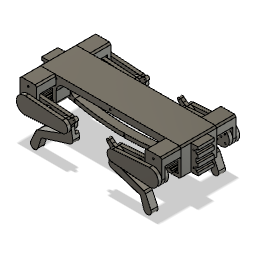
forGazebo v6 (Autodesk Fusion 360 design; units mm, degrees)
Autodesk Fusion 360 part; units mm, degrees
sketch "Sketch1" plane through (0, 0, 0) normal (0, 0, 1) x (1, 0, 0)
  arc A0 (83.6533, -28.925) -> (83.3871, -29.3635) centre (83.6533, -29.225) ccw
  arc A1 (81.6129, -29.3635) -> (83.3871, -29.3635) centre (82.5, -29.825) ccw
  arc A2 (81.6129, -29.3635) -> (81.3467, -28.925) centre (81.3467, -29.225) ccw
  arc A3 (-81.3467, -28.925) -> (-81.6129, -29.3635) centre (-81.3467, -29.225) ccw
  line L0 (-81.3467, -28.925) -> (-79, -28.925)
  arc A4 (-83.3871, -29.3635) -> (-83.6533, -28.925) centre (-83.6533, -29.225) ccw
  line L1 (-86, -28.925) -> (-83.6533, -28.925)
  line L2 (-86, -28.175) -> (-86, -28.925)
  line L3 (-86, -27.675) -> (-86, -28.175)
  line L4 (-79, -28.175) -> (-79, -27.675)
  line L5 (-79, -28.925) -> (-79, -28.175)
  line L6 (79, -28.175) -> (79, -28.925)
  line L7 (79, -27.675) -> (79, -28.175)
  line L8 (83.6533, -28.925) -> (86, -28.925)
  line L9 (86, -28.175) -> (86, -27.675)
  line L10 (86, -28.925) -> (86, -28.175)
  line L11 (79, -28.925) -> (81.3467, -28.925)
  line L12 (-79, -27.675) -> (-77.05, -27.675)
  line L13 (-87.95, -27.675) -> (-86, -27.675)
  line L14 (86, -27.675) -> (87.95, -27.675)
  line L15 (77.05, -27.675) -> (79, -27.675)
  line L16 (102.4, -1.585) -> (100.1, -1.585)
  arc A5 (-83.3871, -29.3635) -> (-81.6129, -29.3635) centre (-82.5, -29.825) ccw
  circle A6 centre (-71.05, 0) radius 1
  circle A7 centre (71.05, 0) radius 1
  circle A8 centre (-65.2986, -31.4552) radius 1
  circle A9 centre (65.2986, -31.4552) radius 1
  circle A10 centre (0, -38.7099) radius 1
  circle A11 centre (-97.3, -24.2) radius 1
  circle A12 centre (-97.3, -4.2) radius 1
  circle A13 centre (97.3, -24.2) radius 1
  circle A14 centre (97.3, -4.2) radius 1
  line L17 (-60, -4.275) -> (-50, -4.275)
  line L18 (-50, 4.275) -> (-60, 4.275)
  line L19 (-85, -4.275) -> (-80, -4.275)
  line L20 (-80, 4.275) -> (-85, 4.275)
  spline S0 degree 3 poles (-83.5, -2.125) (-83.5, -1.9978) (-83.4743, -1.8633) (-83.3718, -1.6174) (-83.2951, -1.5059) (-83.1192, -1.3299) (-83.0076, -1.2532) (-82.7616, -1.1507) (-82.6271, -1.125) (-82.3729, -1.125) (-82.2384, -1.1507) (-81.9924, -1.2532) (-81.8808, -1.3299) (-81.7049, -1.5059) (-81.6282, -1.6174) (-81.5257, -1.8633) (-81.5, -1.9978) (-81.5, -2.2522) (-81.5257, -2.3867) (-81.6282, -2.6326) (-81.7049, -2.7441) (-81.8808, -2.9201) (-81.9924, -2.9968) (-82.2384, -3.0993) (-82.3729, -3.125) (-82.6271, -3.125) (-82.7616, -3.0993) (-83.0076, -2.9968) (-83.1192, -2.9201) (-83.2951, -2.7441) (-83.3718, -2.6326) (-83.4743, -2.3867) (-83.5, -2.2522) (-83.5, -2.125) knots 0 0 0 0 0.038156 0.038156 0.076312 0.076312 0.114429 0.114429 0.152546 0.152546 0.190663 0.190663 0.22878 0.22878 0.266936 0.266936 0.305092 0.305092 0.343248 0.343248 0.381403 0.381403 0.41952 0.41952 0.457638 0.457638 0.495755 0.495755 0.533872 0.533872 0.572028 0.572028 0.610183 0.610183 0.610183 0.610183
  line L21 (80, -4.275) -> (85, -4.275)
  line L22 (85, 4.275) -> (80, 4.275)
  spline S1 degree 3 poles (81.5, -2.125) (81.5, -1.9978) (81.5257, -1.8633) (81.6282, -1.6174) (81.7049, -1.5059) (81.8808, -1.3299) (81.9924, -1.2532) (82.2384, -1.1507) (82.3729, -1.125) (82.6271, -1.125) (82.7616, -1.1507) (83.0076, -1.2532) (83.1192, -1.3299) (83.2951, -1.5059) (83.3718, -1.6174) (83.4743, -1.8633) (83.5, -1.9978) (83.5, -2.2522) (83.4743, -2.3867) (83.3718, -2.6326) (83.2951, -2.7441) (83.1192, -2.9201) (83.0076, -2.9968) (82.7616, -3.0993) (82.6271, -3.125) (82.3729, -3.125) (82.2384, -3.0993) (81.9924, -2.9968) (81.8808, -2.9201) (81.7049, -2.7441) (81.6282, -2.6326) (81.5257, -2.3867) (81.5, -2.2522) (81.5, -2.125) knots 0 0 0 0 0.038156 0.038156 0.076312 0.076312 0.114429 0.114429 0.152546 0.152546 0.190663 0.190663 0.22878 0.22878 0.266936 0.266936 0.305092 0.305092 0.343248 0.343248 0.381403 0.381403 0.41952 0.41952 0.457638 0.457638 0.495755 0.495755 0.533872 0.533872 0.572028 0.572028 0.610183 0.610183 0.610183 0.610183
  line L23 (50, -4.275) -> (60, -4.275)
  line L24 (60, 4.275) -> (50, 4.275)
  line L25 (-85, -4.275) -> (-87.95, -4.275)
  line L26 (80, -4.275) -> (77.05, -4.275)
  line L27 (87.95, -4.275) -> (85, -4.275)
  line L28 (-80, 4.275) -> (-60, 4.275)
  line L29 (-91.5, 4.275) -> (-85, 4.275)
  line L30 (85, 4.275) -> (91.5, 4.275)
  line L31 (60, 4.275) -> (80, 4.275)
  line L32 (-50, 4.275) -> (50, 4.275)
  line L33 (61.05, -4.275) -> (60, -4.275)
  line L34 (-60, -4.275) -> (-61.05, -4.275)
  line L35 (50, -4.275) -> (-50, -4.275)
  circle A15 centre (0, 0) radius 1
  arc A16 (-88.95, -26.675) -> (-87.95, -27.675) centre (-88.95, -27.675) ccw
  arc A17 (-87.95, -4.275) -> (-88.95, -5.275) centre (-88.95, -4.275) ccw
  line L36 (-77.05, -4.275) -> (-80, -4.275)
  arc A18 (-76.05, -5.275) -> (-77.05, -4.275) centre (-76.05, -4.275) ccw
  line L37 (-88.95, -5.275) -> (-88.95, -26.675)
  line L38 (-76.05, -26.675) -> (-76.05, -5.275)
  arc A19 (-77.05, -27.675) -> (-76.05, -26.675) centre (-76.05, -27.675) ccw
  arc A20 (76.05, -26.675) -> (77.05, -27.675) centre (76.05, -27.675) ccw
  arc A21 (77.05, -4.275) -> (76.05, -5.275) centre (76.05, -4.275) ccw
  arc A22 (88.95, -5.275) -> (87.95, -4.275) centre (88.95, -4.275) ccw
  line L39 (76.05, -5.275) -> (76.05, -26.675)
  line L40 (88.95, -26.675) -> (88.95, -5.275)
  arc A23 (87.95, -27.675) -> (88.95, -26.675) centre (88.95, -27.675) ccw
  arc A24 (71.05, -14.275) -> (61.05, -4.275) centre (61.05, -14.275) ccw
  line L41 (71.05, -21.1412) -> (71.05, -14.275)
  arc A25 (64.7498, -29.0162) -> (71.05, -21.1412) centre (62.9781, -21.1412) ccw
  arc A26 (-64.7498, -29.0162) -> (64.7498, -29.0162) centre (0, 258.7901) ccw
  arc A27 (-71.05, -21.1412) -> (-64.7498, -29.0162) centre (-62.9781, -21.1412) ccw
  line L42 (-71.05, -14.275) -> (-71.05, -21.1412)
  arc A28 (-61.05, -4.275) -> (-71.05, -14.275) centre (-61.05, -14.275) ccw
  line L43 (91.5, -32.675) -> (76.8218, -32.675)
  arc A29 (76.8218, -32.675) -> (65.8473, -33.8943) centre (76.8218, -82.675) ccw
  arc A30 (-65.8473, -33.8943) -> (65.8473, -33.8943) centre (0, 258.7901) ccw
  arc A31 (-65.8473, -33.8943) -> (-76.8218, -32.675) centre (-76.8218, -82.675) ccw
  line L44 (-76.8218, -32.675) -> (-91.5, -32.675)
  line L45 (102.9, 2.275) -> (102.9, -1.585)
  line L46 (102.9, -1.585) -> (102.4, -1.585)
  line L47 (93.5, 2.275) -> (102.9, 2.275)
  line L48 (91.5, 4.275) -> (93.5, 2.275)
  line L49 (-93.5, 2.275) -> (-91.5, 4.275)
  line L50 (-102.9, 2.275) -> (-93.5, 2.275)
  line L51 (-102.9, -1.585) -> (-102.9, 2.275)
  line L52 (-100.1, -1.585) -> (-102.9, -1.585)
  line L53 (-100.1, -6.815) -> (-100.1, -1.585)
  line L54 (-102.9, -6.815) -> (-100.1, -6.815)
  line L55 (-102.9, -11.585) -> (-102.9, -6.815)
  line L56 (-100.1, -11.585) -> (-102.9, -11.585)
  line L57 (-100.1, -16.815) -> (-100.1, -11.585)
  line L58 (-102.9, -16.815) -> (-100.1, -16.815)
  line L59 (-102.9, -21.585) -> (-102.9, -16.815)
  line L60 (-100.1, -21.585) -> (-102.9, -21.585)
  line L61 (-100.1, -26.815) -> (-100.1, -21.585)
  line L62 (-102.9, -26.815) -> (-100.1, -26.815)
  line L63 (-102.9, -30.675) -> (-102.9, -26.815)
  line L64 (-93.5, -30.675) -> (-102.9, -30.675)
  line L65 (-91.5, -32.675) -> (-93.5, -30.675)
  line L66 (93.5, -30.675) -> (91.5, -32.675)
  line L67 (102.9, -30.675) -> (93.5, -30.675)
  line L68 (102.9, -26.815) -> (102.9, -30.675)
  line L69 (100.1, -26.815) -> (102.9, -26.815)
  line L70 (100.1, -21.585) -> (100.1, -26.815)
  line L71 (102.9, -21.585) -> (100.1, -21.585)
  line L72 (102.9, -16.815) -> (102.9, -21.585)
  line L73 (100.1, -16.815) -> (102.9, -16.815)
  line L74 (100.1, -11.585) -> (100.1, -16.815)
  line L75 (102.9, -11.585) -> (100.1, -11.585)
  line L76 (102.9, -6.815) -> (102.9, -11.585)
  line L77 (100.1, -6.815) -> (102.9, -6.815)
  line L78 (100.1, -1.585) -> (100.1, -6.815)
  arc A32 (-81.3467, -28.925) -> (-81.6129, -29.3635) centre (-81.3467, -29.225) ccw
  arc A33 (-83.3871, -29.3635) -> (-81.6129, -29.3635) centre (-82.5, -29.825) ccw
  arc A34 (-83.3871, -29.3635) -> (-83.6533, -28.925) centre (-83.6533, -29.225) ccw
  line L79 (-83.6533, -28.925) -> (-86, -28.925)
  line L80 (-86, -28.925) -> (-86, -27.675)
  line L81 (-86, -27.675) -> (-87.95, -27.675)
  arc A35 (-88.95, -26.675) -> (-87.95, -27.675) centre (-88.95, -27.675) ccw
  line L82 (-88.95, -26.675) -> (-88.95, -5.275)
  arc A36 (-87.95, -4.275) -> (-88.95, -5.275) centre (-88.95, -4.275) ccw
  line L83 (-87.95, -4.275) -> (-77.05, -4.275)
  arc A37 (-76.05, -5.275) -> (-77.05, -4.275) centre (-76.05, -4.275) ccw
  line L84 (-76.05, -5.275) -> (-76.05, -26.675)
  arc A38 (-77.05, -27.675) -> (-76.05, -26.675) centre (-76.05, -27.675) ccw
  line L85 (-77.05, -27.675) -> (-79, -27.675)
  line L86 (-79, -27.675) -> (-79, -28.925)
  line L87 (-79, -28.925) -> (-81.3467, -28.925)
  arc A39 (83.6533, -28.925) -> (83.3871, -29.3635) centre (83.6533, -29.225) ccw
  arc A40 (81.6129, -29.3635) -> (83.3871, -29.3635) centre (82.5, -29.825) ccw
  arc A41 (81.6129, -29.3635) -> (81.3467, -28.925) centre (81.3467, -29.225) ccw
  line L88 (81.3467, -28.925) -> (79, -28.925)
  line L89 (79, -28.925) -> (79, -27.675)
  line L90 (79, -27.675) -> (77.05, -27.675)
  arc A42 (76.05, -26.675) -> (77.05, -27.675) centre (76.05, -27.675) ccw
  line L91 (76.05, -26.675) -> (76.05, -5.275)
  arc A43 (77.05, -4.275) -> (76.05, -5.275) centre (76.05, -4.275) ccw
  line L92 (77.05, -4.275) -> (87.95, -4.275)
  arc A44 (88.95, -5.275) -> (87.95, -4.275) centre (88.95, -4.275) ccw
  line L93 (88.95, -5.275) -> (88.95, -26.675)
  arc A45 (87.95, -27.675) -> (88.95, -26.675) centre (88.95, -27.675) ccw
  line L94 (87.95, -27.675) -> (86, -27.675)
  line L95 (86, -27.675) -> (86, -28.925)
  line L96 (86, -28.925) -> (83.6533, -28.925)
  circle A46 centre (0, 0) radius 1
  circle A47 centre (71.05, 0) radius 1
  circle A48 centre (-71.05, 0) radius 1
  line L97 (91.5, -32.675) -> (93.5, -30.675)
  line L98 (93.5, -30.675) -> (93.5, 2.275)
  line L99 (93.5, 2.275) -> (91.5, 4.275)
  line L100 (91.5, 4.275) -> (-91.5, 4.275)
  line L101 (-91.5, 4.275) -> (-93.5, 2.275)
  line L102 (-93.5, 2.275) -> (-93.5, -30.675)
  line L103 (-93.5, -30.675) -> (-91.5, -32.675)
  line L104 (-91.5, -32.675) -> (-76.8218, -32.675)
  arc A49 (-76.1202, -32.6799) -> (-76.8218, -32.675) centre (-76.8218, -82.675) ccw
  arc A50 (-76.1202, -32.6799) -> (-71.05, -27.6804) centre (-76.05, -27.6804) ccw
  line L105 (-71.05, -27.6804) -> (-71.05, -14.275)
  arc A51 (-61.05, -4.275) -> (-71.05, -14.275) centre (-61.05, -14.275) ccw
  line L106 (-61.05, -4.275) -> (61.05, -4.275)
  arc A52 (71.05, -14.275) -> (61.05, -4.275) centre (61.05, -14.275) ccw
  line L107 (71.05, -14.275) -> (71.05, -27.6804)
  arc A53 (71.05, -27.6804) -> (76.1202, -32.6799) centre (76.05, -27.6804) ccw
  arc A54 (76.8218, -32.675) -> (76.1202, -32.6799) centre (76.8218, -82.675) ccw
  line L108 (76.8218, -32.675) -> (91.5, -32.675)
  circle A55 centre (-82.5, -2.125) radius 1
  circle A56 centre (82.5, -2.125) radius 1
extrude "Extrude1" add sketch "Sketch1" along normal mid plane 47 contours L17 L18 L20 L22 L23 L24 L28 L29 L30 L31 L32 L33 L34 L35 A24 L41 L42 A28 L43 A29 A31 L44 L48 L49 L65 L66 L97 L98 L99 L100 L101 L102 L103 L104 A49 A50 L105 A51 L106 A52 L107 A53 A54 L108 makes body 1
extrude "Extrude2" add sketch "Sketch1" along normal mid plane 10 contours A25 A26 A27 A29 A30 A31 A50 L105 L107 A53 bodies 1
extrude "Extrude3" add sketch "Sketch1" along normal mid plane 21.2 contours L16 L45 L46 L47 L67 L68 L69 L70 L71 L72 L73 L74 L75 L76 L77 L78 L98 | L50 L51 L52 L53 L54 L55 L56 L57 L58 L59 L60 L61 L62 L63 L64 L102 bodies 1
sketch "Sketch2" plane through (0, 0, 0) normal (0, 0, 1) x (1, 0, 0)
  arc A0 (6.5, 11.2583) -> (-6.5, 11.2583) centre (0, 0) ccw
  arc A1 (6.5, 11.2583) -> (11, 13.8564) centre (8, 13.8564) ccw
  line L0 (11, 13.8564) -> (11, 0)
  arc A2 (-11, 0) -> (11, 0) centre (0, 0) ccw
  line L1 (-11, 0) -> (-11, 13.8564)
  arc A3 (-11, 13.8564) -> (-6.5, 11.2583) centre (-8, 13.8564) ccw
  circle A4 centre (0, 0) radius 5.2
  line L2 (-6.45, 15.8143) -> (-6.45, 11.2871)
  arc A5 (-6.45, 11.2871) -> (-6.5, 11.2583) centre (0, 0.0004) ccw
  arc A6 (-11, 13.8564) -> (-6.5, 11.2583) centre (-8, 13.8564) ccw
  line L3 (-11, 13.8564) -> (-11, 23.5)
  line L4 (-11, 23.5) -> (-9, 25.5)
  line L5 (-9, 25.5) -> (9, 25.5)
  line L6 (9, 25.5) -> (11, 23.5)
  line L7 (11, 23.5) -> (11, 13.8564)
  arc A7 (6.5, 11.2583) -> (11, 13.8564) centre (8, 13.8564) ccw
  arc A8 (6.5, 11.2583) -> (6.45, 11.2871) centre (0, 0.0004) ccw
  line L8 (6.45, 11.2871) -> (6.45, 15.8143)
  arc A9 (6.45, 15.8143) -> (6.45, 17.7928) centre (6.3036, 16.8036) ccw
  line L9 (6.45, 17.7928) -> (6.45, 20.7)
  arc A10 (6.45, 20.7) -> (5.45, 21.7) centre (6.45, 21.7) ccw
  line L10 (5.45, 21.7) -> (-5.45, 21.7)
  arc A11 (-5.45, 21.7) -> (-6.45, 20.7) centre (-6.45, 21.7) ccw
  line L11 (-6.45, 20.7) -> (-6.45, 17.7928)
  arc A12 (-6.45, 17.7928) -> (-6.45, 15.8143) centre (-6.3036, 16.8036) ccw
  circle A13 centre (0, 19.1) radius 1.1
  arc A14 (6.45, 20.7) -> (5.45, 21.7) centre (6.45, 21.7) ccw
  line L12 (6.45, 20.7) -> (6.45, 17.7928)
  arc A15 (6.45, 17.7928) -> (5.3143, 16.95) centre (6.3036, 16.8036) ccw
  line L13 (5.3143, 16.95) -> (-5.3143, 16.95)
  arc A16 (-5.3143, 16.95) -> (-6.45, 17.7928) centre (-6.3036, 16.8036) ccw
  line L14 (-6.45, 17.7928) -> (-6.45, 20.7)
  arc A17 (-5.45, 21.7) -> (-6.45, 20.7) centre (-6.45, 21.7) ccw
  line L15 (-5.45, 21.7) -> (5.45, 21.7)
  arc A18 (6.45, 15.8143) -> (5.3143, 16.95) centre (6.3036, 16.8036) ccw
  line L16 (6.45, 15.8143) -> (6.45, 11.2871)
  arc A19 (6.45, 11.2871) -> (-6.45, 11.2871) centre (0, 0) ccw
  line L17 (-6.45, 11.2871) -> (-6.45, 15.8143)
  arc A20 (-5.3143, 16.95) -> (-6.45, 15.8143) centre (-6.3036, 16.8036) ccw
  line L18 (-5.3143, 16.95) -> (5.3143, 16.95)
extrude "Extrude4" add sketch "Sketch2" along normal blind 4.3 separate body contours A0 A1 L0 A2 L1 A3 A5 A6 A7 A8 A19 makes body 2
extrude "Extrude8" add sketch "Sketch2" along normal blind 25.45 contours A0 A1 A3 L2 A5 A6 L3 L4 L5 L6 L7 A7 A8 L8 A9 L9 A10 L10 A11 L11 A12 A14 L12 L14 A17 L15 A18 L16 L17 A20 | A0 L2 L8 A9 A12 A15 L13 A16 A18 L16 A19 L17 A20 L18 | L9 A10 L10 A11 L11 A14 L12 A15 L13 A16 L14 A17 L15 A18 A20 L18 bodies 2
sketch "Sketch3" plane through (0, 0, 0) normal (0, 0, 1) x (1, 0, 0)
  arc A0 (-2.3695, -9.1998) -> (5.814, -7.5131) centre (0, 0) ccw
  arc A1 (-2.3695, -9.1998) -> (-4.7523, -10.4653) centre (-2.8683, -11.1366) ccw
  arc A2 (-4.7523, -10.4653) -> (-5.062, -6.4127) centre (-9.4622, -8.7871) ccw
  line L0 (-5.062, -6.4127) -> (-6.6004, -3.5615)
  arc A3 (0.3966, 7.4895) -> (-6.6004, -3.5615) centre (0, 0) ccw
  arc A4 (0.3966, 7.4895) -> (5.5943, 9.2171) centre (0.7933, 14.979) ccw
  line L1 (5.5943, 9.2171) -> (8.8728, 11.9488)
  arc A5 (12.3225, 8.346) -> (8.8728, 11.9488) centre (10.5242, 10.0771) ccw
  line L2 (12.3225, 8.346) -> (9.4511, 5.1891)
  arc A6 (9.4511, 5.1891) -> (7.5099, 0.5399) centre (14.9993, 0.1426) ccw
  line L3 (7.5099, 0.5399) -> (9.0125, -8.7764)
  arc A7 (9.0125, -8.7764) -> (5.814, -7.5131) centre (7.038, -9.0949) ccw
  circle A8 centre (0, 0) radius 5.2
  circle A9 centre (10.4731, 10.0281) radius 0.5
  arc A10 (-2.3695, -9.1998) -> (-4.7523, -10.4653) centre (-2.8683, -11.1366) ccw
  arc A11 (-2.3695, -9.1998) -> (5.814, -7.5131) centre (0, 0) ccw
  arc A12 (9.0125, -8.7764) -> (5.814, -7.5131) centre (7.038, -9.0949) ccw
  line L4 (9.0125, -8.7764) -> (9.7594, -13.4072)
  arc A13 (6.3178, -18.9748) -> (9.7594, -13.4072) centre (4.8232, -14.2034) ccw
  line L5 (6.3178, -18.9748) -> (-31.7747, -30.9066)
  line L6 (-31.7747, -30.9066) -> (-36.3472, -45.0876)
  arc A14 (-45.6515, -41.4706) -> (-36.3472, -45.0876) centre (-41.1059, -43.5533) ccw
  line L7 (-45.6515, -41.4706) -> (-38.5828, -26.0423)
  arc A15 (-36.3223, -23.9525) -> (-38.5828, -26.0423) centre (-34.9463, -27.7084) ccw
  line L8 (-36.3223, -23.9525) -> (-7.7422, -13.4819)
  arc A16 (-7.7422, -13.4819) -> (-4.7523, -10.4653) centre (-9.4622, -8.7871) ccw
extrude "Extrude9" add sketch "Sketch3" along normal blind 4.3 separate body contours A0 A1 A2 L0 A3 A4 L1 A5 L2 A6 L3 A7 A10 A11 A12 makes body 3
extrude "Extrude10" add sketch "Sketch3" along normal blind 8.9 contours A0 A1 A7 A10 A11 A12 L4 A13 L5 L6 A14 L7 A15 L8 A16 bodies 3
sketch "Sketch4" plane through (0, 0, 0) normal (0, 0, 1) x (1, 0, 0)
  circle A0 centre (-27.389, -5.2162) radius 1.1
  circle A1 centre (-27.2162, 5.389) radius 1.1
  circle A2 centre (-16.611, 5.2162) radius 1.1
  circle A3 centre (-16.7838, -5.389) radius 1.1
  circle A4 centre (-22, 0) radius 1
  circle A5 centre (27, 0) radius 1
  circle A6 centre (-8.6, 0) radius 1
  circle A7 centre (19.1, 0) radius 1
  arc A8 (5.7098, -3.0001) -> (5.7098, 3.0001) centre (5.6493, 0) ccw
  arc A9 (5.7098, 3.0001) -> (5.7098, -3.0001) centre (0, 0) ccw
  arc A10 (-21.2143, 10.9719) -> (-21.2143, -10.9719) centre (-22, 0) ccw
  line L0 (-21.2143, 10.9719) -> (27.5357, 7.4808)
  arc A11 (27.5357, -7.4808) -> (27.5357, 7.4808) centre (27, 0) ccw
  line L1 (27.5357, -7.4808) -> (-21.2143, -10.9719)
  circle A12 centre (-22, 0) radius 1
  circle A13 centre (-22, 0) radius 5
  circle A14 centre (27, 0) radius 1
  circle A15 centre (27, 0) radius 5
extrude "Extrude11" add sketch "Sketch4" along normal blind 4.5 separate body contours A10 L0 A11 L1 makes body 4
extrude "Extrude12" add sketch "Sketch4" along normal blind 11 contours A13 | A15 bodies 4
sketch "Sketch5" plane through (0, 0, 0) normal (0, 0, 1) x (1, 0, 0)
  arc A0 (36.1636, 4.1203) -> (30.7636, 4.1203) centre (33.4636, 4.1203) ccw
  line L0 (30.7636, 4.1203) -> (30.7636, -4.1203)
  arc A1 (30.7636, -4.1203) -> (36.1636, -4.1203) centre (33.4636, -4.1203) ccw
  line L1 (36.1636, -4.1203) -> (36.1636, 4.1203)
  circle A2 centre (49, 0) radius 5.2
  circle A3 centre (0, 0) radius 5.2
  line L2 (0.7857, 10.9719) -> (49.5357, 7.4808)
  arc A4 (49.5357, -7.4808) -> (49.5357, 7.4808) centre (49, 0) ccw
  line L3 (49.5357, -7.4808) -> (0.7857, -10.9719)
  arc A5 (0.7857, 10.9719) -> (0.7857, -10.9719) centre (0, 0) ccw
extrude "Extrude13" add sketch "Sketch5" along normal blind 4.5 separate body contours A0 L0 A1 L1 | L2 A4 L3 A5 makes body 5
extrude "Extrude14" add sketch "Sketch5" along normal blind 2.5 contours A2 | A3 bodies 5
copy_body "CopyPasteBodies8" bodies 5 makes body 6
copy_body "CopyPasteBodies9" bodies 5 makes body 7
copy_body "CopyPasteBodies10" bodies 5 makes body 8
copy_body "CopyPasteBodies1" bodies 4 makes body 9
copy_body "CopyPasteBodies2" bodies 4 makes body 10
copy_body "CopyPasteBodies3" bodies 4 makes body 11
mirror "Mirror1" about plane through (0, 0, 0) normal (1, 0, 0) of bodies 3 makes body 12
copy_body "CopyPasteBodies4" bodies 12 3 makes body 13 makes body 14
copy_body "CopyPasteBodies5" bodies 2 makes body 15
copy_body "CopyPasteBodies6" bodies 2 makes body 16
copy_body "CopyPasteBodies7" bodies 2 makes body 17
move_body "Move1" bodies 2 to x (1, 0, 0) y (0, 1, 0) z (0, 0, 1) at (55, 0, -70)
move_body "Move2" bodies 15 to x (1, 0, 0) y (0, 1, 0) z (0, 0, 1) at (0, 0, 65)
move_body "Move3" bodies 15 to x (-1, 0, 0) y (0, 1, 0) z (0, 0, -1) at (53, 0, 145)
move_body "Move4" bodies 16 to x (1, 0, 0) y (0, 1, 0) z (0, 0, 1) at (-80, 0, -80)
move_body "Move5" bodies 17 to x (-1, 0, 0) y (0, 1, 0) z (0, 0, -1) at (-22, -82.2335, 78.7873)
move_body "Move6" bodies 3 to x (1, 0, 0) y (0, 1, 0) z (0, 0, 1) at (0, -44.3808, -119.7428)
move_body "Move7" bodies 4 to x (1, 0, 0) y (0, 1, 0) z (0, 0, 1) at (0, -65.5777, -156.5334)
move_body "Move8" bodies 9 to x (1, 0, 0) y (0, 1, 0) z (0, 0, 1) at (0, -84.7944, 135.0144)
move_body "Move9" bodies 4 to x (-1, 0, 0) y (0, 1, 0) z (0, 0, -1) at (19.8475, 0, -291.5563)
move_body "Move10" bodies 10 to x (1, 0, 0) y (0, 1, 0) z (0, 0, 1) at (0, 58.139, 143.3443)
move_body "Move11" bodies 11 to x (-1, 0, 0) y (0, 1, 0) z (0, 0, -1) at (76.2421, 0, -132.3101)
move_body "Move12" bodies 12 to x (1, 0, 0) y (0, 1, 0) z (0, 0, 1) at (0, 79.2326, -103.7771)
move_body "Move13" bodies 13 to x (-1, 0, 0) y (0, 1, 0) z (0, 0, -1) at (-50.0021, -8.4048, 113.7563)
move_body "Move14" bodies 14 to x (-1, 0, 0) y (0, 1, 0) z (0, 0, -1) at (-27.1152, 78.0321, 117.3447)
copy_body "Body->Comp1" bodies 1 removing the originals makes body 18 in component "old_component"
copy_body "Body->Comp2" bodies 9 removing the originals makes body 19 in component "old_component (1)"
copy_body "Body->Comp3" bodies 16 removing the originals makes body 20 in component "old_component (2)"
copy_body "Body->Comp4" bodies 17 removing the originals makes body 21 in component "old_component (3)"
copy_body "Body->Comp5" bodies 15 removing the originals makes body 22 in component "old_component (4)"
copy_body "Body->Comp6" bodies 4 removing the originals makes body 23 in component "old_component (5)"
copy_body "Body->Comp7" bodies 12 removing the originals makes body 24 in component "old_component (6)"
copy_body "Body->Comp8" bodies 14 removing the originals makes body 25 in component "old_component (7)"
copy_body "Body->Comp9" bodies 10 removing the originals makes body 26 in component "old_component (8)"
copy_body "Body->Comp10" bodies 11 removing the originals makes body 27 in component "old_component (9)"
copy_body "Body->Comp11" bodies 13 removing the originals makes body 28 in component "old_component (10)"
copy_body "Body->Comp12" bodies 2 removing the originals makes body 29 in component "old_component (11)"
copy_body "Body->Comp13" bodies 3 removing the originals makes body 30 in component "old_component (12)"
copy_body "Body->Comp14" bodies 5 removing the originals makes body 31 in component "old_component (13)"
copy_body "Body->Comp15" bodies 7 removing the originals makes body 32 in component "old_component (14)"
copy_body "Body->Comp16" bodies 6 removing the originals makes body 33 in component "old_component (15)"
copy_body "Body->Comp17" bodies 8 removing the originals makes body 34 in component "old_component (16)"
copy_body "CopyPasteBodies1'" bodies 18 body 18 seen with x (1, 0, 0) y (0, 1, 0) z (0, 0, 1) at (0, -4.275, 0) makes body 35 in component "base_link"
copy_body "CopyPasteBodies1''" bodies 19 body 19 seen with x (-1, 0, 0) y (0, -1, 0) z (0, 0, 1) at (60.5, -110.2944, -94.9644) makes body 36 in component "forearm_4_1"
copy_body "CopyPasteBodies1'''" bodies 20 body 20 seen with x (1, 0, 0) y (0, 1, 0) z (0, 0, 1) at (-2.5, -25.5, 31.05) makes body 37 in component "shoulder_3_1"
copy_body "CopyPasteBodies1''''" bodies 21 body 21 seen with x (1, 0, 0) y (0, 1, 0) z (0, 0, 1) at (-60.5, 56.7335, -29.8373) makes body 38 in component "shoulder_4_1"
copy_body "CopyPasteBodies1'''''" bodies 22 body 22 seen with x (1, 0, 0) y (0, 1, 0) z (0, 0, 1) at (29.5, -25.5, -31.05) makes body 39 in component "shoulder_2_1"
copy_body "CopyPasteBodies1''''''" bodies 23 body 23 seen with x (-1, 0, 0) y (0, -1, 0) z (0, 0, 1) at (-40.6525, -91.0777, 94.9729) makes body 40 in component "forearm_3_1"
copy_body "CopyPasteBodies1'''''''" bodies 24 body 24 seen with x (1, 0, 0) y (0, 1, 0) z (0, 0, 1) at (33.5, -104.7326, 54.8271) makes body 41 in component "leg_1_1"
copy_body "CopyPasteBodies1''''''''" bodies 25 body 25 seen with x (1, 0, 0) y (0, 1, 0) z (0, 0, 1) at (60.6152, -103.5321, -68.3947) makes body 42 in component "leg_2_1"
copy_body "CopyPasteBodies1'''''''''" bodies 26 body 26 seen with x (1, 0, 0) y (0, 1, 0) z (0, 0, 1) at (-60.5, -83.639, -103.2943) makes body 43 in component "forearm_2_1"
copy_body "CopyPasteBodies1''''''''''" bodies 27 body 27 seen with x (1, 0, 0) y (0, 1, 0) z (0, 0, 1) at (-15.7421, -25.5, 92.2601) makes body 44 in component "forearm_1_1"
copy_body "CopyPasteBodies1'''''''''''" bodies 28 body 28 seen with x (1, 0, 0) y (0, 1, 0) z (0, 0, 1) at (16.5021, -17.0952, -64.8063) makes body 45 in component "leg_4_1"
copy_body "CopyPasteBodies1''''''''''''" bodies 29 body 29 seen with x (1, 0, 0) y (0, 1, 0) z (0, 0, 1) at (27.5, -25.5, 21.05) makes body 46 in component "shoulder_1_1"
copy_body "CopyPasteBodies1'''''''''''''" bodies 30 body 30 seen with x (1, 0, 0) y (0, 1, 0) z (0, 0, 1) at (-33.5, 18.8808, 70.7928) makes body 47 in component "leg_3_1"
copy_body "CopyPasteBodies1''''''''''''''" bodies 31 body 31 seen with x (-1, 0, 0) y (0, 1, 0) z (0, 0, -1) at (82.5, -25.5, 53.55) makes body 48 in component "cover_1_1"
copy_body "CopyPasteBodies1'''''''''''''''" bodies 32 body 32 seen with x (1, 0, 0) y (0, 1, 0) z (0, 0, 1) at (-82.5, -25.5, -53.55) makes body 49 in component "cover_3_1"
copy_body "CopyPasteBodies1''''''''''''''''" bodies 33 body 33 seen with x (-1, 0, 0) y (0, -1, 0) z (0, 0, 1) at (82.5, -25.5, -53.55) makes body 50 in component "cover_2_1"
copy_body "CopyPasteBodies1'''''''''''''''''" bodies 34 body 34 seen with x (1, 0, 0) y (0, -1, 0) z (0, 0, -1) at (-82.5, -25.5, 53.55) makes body 51 in component "cover_4_1"
component "old_component" placed x (1, 0, 0) y (0, 1, 0) z (0, 0, 1) at (0, -4.275, 0)
component "old_component (1)" placed x (-1, 0, 0) y (0, -1, 0) z (0, 0, 1) at (60.5, -110.2944, -94.9644)
component "old_component (2)" placed x (1, 0, 0) y (0, 1, 0) z (0, 0, 1) at (-2.5, -25.5, 31.05)
component "old_component (3)" placed x (1, 0, 0) y (0, 1, 0) z (0, 0, 1) at (-60.5, 56.7335, -29.8373)
component "old_component (4)" placed x (1, 0, 0) y (0, 1, 0) z (0, 0, 1) at (29.5, -25.5, -31.05)
component "old_component (5)" placed x (-1, 0, 0) y (0, -1, 0) z (0, 0, 1) at (-40.6525, -91.0777, 94.9729)
component "old_component (6)" placed x (1, 0, 0) y (0, 1, 0) z (0, 0, 1) at (33.5, -104.7326, 54.8271)
component "old_component (7)" placed x (1, 0, 0) y (0, 1, 0) z (0, 0, 1) at (60.6152, -103.5321, -68.3947)
component "old_component (8)" placed x (1, 0, 0) y (0, 1, 0) z (0, 0, 1) at (-60.5, -83.639, -103.2943)
component "old_component (9)" placed x (1, 0, 0) y (0, 1, 0) z (0, 0, 1) at (-15.7421, -25.5, 92.2601)
component "old_component (10)" placed x (1, 0, 0) y (0, 1, 0) z (0, 0, 1) at (16.5021, -17.0952, -64.8063)
component "old_component (11)" placed x (1, 0, 0) y (0, 1, 0) z (0, 0, 1) at (27.5, -25.5, 21.05)
component "old_component (12)" placed x (1, 0, 0) y (0, 1, 0) z (0, 0, 1) at (-33.5, 18.8808, 70.7928)
component "old_component (13)" placed x (-1, 0, 0) y (0, 1, 0) z (0, 0, -1) at (82.5, -25.5, 53.55)
component "old_component (14)" placed x (1, 0, 0) y (0, 1, 0) z (0, 0, 1) at (-82.5, -25.5, -53.55)
component "old_component (15)" placed x (-1, 0, 0) y (0, -1, 0) z (0, 0, 1) at (82.5, -25.5, -53.55)
component "old_component (16)" placed x (1, 0, 0) y (0, -1, 0) z (0, 0, -1) at (-82.5, -25.5, 53.55)
component "base_link" placed x (1, 0, 0) y (0, 1, 0) z (0, 0, 1) at (0, 0, 0)
component "forearm_4_1" placed x (1, 0, 0) y (0, 1, 0) z (0, 0, 1) at (0, 0, 0)
component "shoulder_3_1" placed x (1, 0, 0) y (0, 1, 0) z (0, 0, 1) at (0, 0, 0)
component "shoulder_4_1" placed x (1, 0, 0) y (0, 1, 0) z (0, 0, 1) at (0, 0, 0)
component "shoulder_2_1" placed x (1, 0, 0) y (0, 1, 0) z (0, 0, 1) at (0, 0, 0)
component "forearm_3_1" placed x (1, 0, 0) y (0, 1, 0) z (0, 0, 1) at (0, 0, 0)
component "leg_1_1" placed x (1, 0, 0) y (0, 1, 0) z (0, 0, 1) at (0, 0, 0)
component "leg_2_1" placed x (1, 0, 0) y (0, 1, 0) z (0, 0, 1) at (0, 0, 0)
component "forearm_2_1" placed x (1, 0, 0) y (0, 1, 0) z (0, 0, 1) at (0, 0, 0)
component "forearm_1_1" placed x (1, 0, 0) y (0, 1, 0) z (0, 0, 1) at (0, 0, 0)
component "leg_4_1" placed x (1, 0, 0) y (0, 1, 0) z (0, 0, 1) at (0, 0, 0)
component "shoulder_1_1" placed x (1, 0, 0) y (0, 1, 0) z (0, 0, 1) at (0, 0, 0)
component "leg_3_1" placed x (1, 0, 0) y (0, 1, 0) z (0, 0, 1) at (0, 0, 0)
component "cover_1_1" placed x (1, 0, 0) y (0, 1, 0) z (0, 0, 1) at (0, 0, 0)
component "cover_3_1" placed x (1, 0, 0) y (0, 1, 0) z (0, 0, 1) at (0, 0, 0)
component "cover_2_1" placed x (1, 0, 0) y (0, 1, 0) z (0, 0, 1) at (0, 0, 0)
component "cover_4_1" placed x (1, 0, 0) y (0, 1, 0) z (0, 0, 1) at (0, 0, 0)
named bodies: "base_link", "shoulder_1", "leg_3", "forearm_3", "forearm_4", "forearm_2", "forearm_1", "leg_1", "leg_4", "leg_2", "shoulder_2", "shoulder_3", "shoulder_4", "cover_1", "cover", "cover_2", "cover (1)", "cover_3", "cover (2)", "cover_4"
